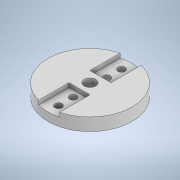
# Autodesk Inventor part: prop_retaining_part
Saved by Autodesk Inventor 2021 (Build 250183000, 183)
## iProperties
Created: 2020-08-19
Part Number: prop_retaining_part
Material: Generic
Document SubType Name: Modeling
Designer: elizabethhassan
Density: 1 g/cm^3
Appearance: Default
Author: elizabethhassan
Autodesk Inventor part; units mm, degrees
ref_plane "YZ Plane" through (0, 0, 0) normal (1, 0, 0) x (0, 1, 0)
ref_plane "XZ Plane" through (0, 0, 0) normal (0, 1, 0) x (-1, 0, 0)
ref_plane "XY Plane" through (0, 0, 0) normal (0, 0, 1) x (1, 0, 0)
sketch "Sketch1" plane through (0, 0, 0) normal (0, 1, 0) x (-1, 0, 0)
  circle A0 centre (0, 0) radius 20
  dimension "d0" = 40
  constraints: 1 centre point, 1 coincident
  measures "d0" diameter of A0
extrude "Extrusion1" add sketch "Sketch1" along normal blind 6
sketch "Sketch3" plane through (0, 6, 0) normal (0, 1, 0) x (1, 0, 0)
  line L0 (0, 0) -> (0, 20)
  circle A0 centre (0, 0) radius 20 projected
  line L1 (5, 35) -> (5, 5)
  line L2 (5, 5) -> (-5, 5)
  line L3 (-5, 5) -> (-5, 35)
  line L4 (-5, 35) -> (5, 35)
  line L5 (5, 35) -> (-5, 5) construction
  line L6 (5, 5) -> (-5, 35) construction
  line L7 (20, 0) -> (-20, 0) construction
  line L8 (5, -35) -> (5, -5)
  line L9 (5, -5) -> (-5, -5)
  line L10 (-5, -5) -> (-5, -35)
  line L11 (-5, -35) -> (5, -35)
  point P0 (-5, 19.3649)
  point P1 (5, 19.3649)
  point P2 (-5, -19.3649)
  point P3 (5, -19.3649)
  dimension "d11" = 30
  dimension "d12" = 10
  constraints: 24 end point, 4 symmetric about line, 3 point on circle, 2 midpoint, 2 parallel, 1 horizontal, 1 perpendicular, 1 vertical
  measures "d11" distance of L1.start L1.end
  measures "d12" distance of L1.end L2.end
extrude "Extrusion2" cut sketch "Sketch3" against normal blind 2 contours L2 L3 A0 L0 | L0 A0 L1 L2 | L10 L9 L8 A0
sketch "Sketch5" plane through (0, 4, 0) normal (0, 1, 0) x (1, 0, 0)
  circle A0 centre (0, -8) radius 1
  circle A1 centre (0, -15) radius 1
  line L0 (-5, -5) -> (5, -5) projected
  arc A2 (-5, 19.3649) -> (-5, -19.3649) centre (0, 0) ccw projected
  line L1 (-20, 0) -> (20, 0) construction
  arc A3 (5, -19.3649) -> (5, 19.3649) centre (0, 0) ccw projected
  circle A4 centre (0, 8) radius 1
  circle A5 centre (0, 15) radius 1
  line L2 (5, 5) -> (-5, 5) projected
  line L3 (5, 19.3649) -> (5, 5) projected
  dimension "d20" = 2
  dimension "d21" = 2
  dimension "d22" = 3
  dimension "d23" = 7
  dimension "d39" = 3
  dimension "d40" = 5
  dimension "d41" = 5
  constraints: 4 centre point, 2 end point, 2 point on circle, 2 symmetric about line, 1 horizontal, 2 other
  measures "d20" diameter of A0
  measures "d21" diameter of A1
  measures "d22" distance from line of A0.centre L0
  measures "d23" distance of A1.centre A0.centre
  measures "d39" distance from line of A4.centre L2
  measures "d40" distance from line of L3 A4.centre
  measures "d41" distance from line of L3 A5.centre
hole "Hole2" at (0, 4, 15) at (0, 4, 8) at (0, 4, -8) at (0, 4, -15) direction (0, -1, 0) diameter 3.4 depth 10.979 tip angle 118 clearance for "Flat Head Machine Screw" size "M3" standard "Ansi Metric M Profile"
sketch "Sketch6" plane through (0, 0, 0) normal (0, -1, 0) x (1, 0, 0)
  circle A0 centre (0, 0) radius 1.5
  dimension "d31" = 3
  constraints: 1 centre point, 1 coincident
  measures "d31" diameter of A0
hole "Hole3" at (0, 0, 0) direction (0, 1, 0) diameter 5.5 depth 8.8 tip angle 118 countersink diameter 6.8 countersink angle 90 clearance for "Flat Head Machine Screw" size "M5" standard "Ansi Metric M Profile"
body "Solid1"
